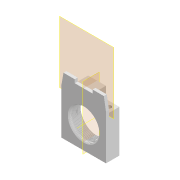
# Autodesk Inventor part: 30_Cube_Z_Focus_MGN_NEMA_adapter_RMS_bolted
Saved by Autodesk Inventor 2022 (Build 260153000, 153)
## iProperties
Created: 2021-04-25
Part Number: 30_Cube_Z_Focus_MGN_NEMA_adapter_RMS_bolted
Material: Generic
Document SubType Name: Modeling
Designer: diederichbenedict
Density: 1 g/cm^3
Appearance: Default
Author: diederichbenedict
Autodesk Inventor part; units mm, degrees
ref_plane "YZ Plane" through (0, 0, 0) normal (1, 0, 0) x (0, 1, 0)
ref_plane "XZ Plane" through (0, 0, 0) normal (0, 1, 0) x (-1, 0, 0)
ref_plane "XY Plane" through (0, 0, 0) normal (0, 0, 1) x (1, 0, 0)
ref_plane "Work Plane1" through (0, 0, 0) normal (0, 0, 1) x (1, 0, 0)
sketch "Sketch1" plane through (0, 0, 0) normal (0, 0, 1) x (1, 0, 0)
  circle A0 centre (6.843, -28.9967) radius 1.4 projected
  circle A1 centre (26.1569, -28.9967) radius 1.4 projected
  circle A2 centre (26.1569, -23.9967) radius 1.4 projected
  circle A3 centre (6.843, -23.9967) radius 1.4 projected
  line L0 (0.4643, -12) -> (0, -12) construction
  line L1 (3.1567, -14.6923) -> (0.4643, -12) construction
  line L2 (3.1567, -32.6831) -> (3.1567, -14.6923) construction
  line L3 (10.5294, -32.6831) -> (3.1567, -32.6831) projected
  line L4 (10.5294, -14.6923) -> (10.5294, -32.6831) construction
  line L5 (9, -11) -> (10.5294, -14.6923) construction
  line L6 (2.8, -11) -> (9, -11) construction
  line L7 (2.8, 0) -> (2.8, -11) construction
  line L8 (30.2, 0) -> (2.8, 0) construction
  line L9 (30.2, 0) -> (30.2, -11) construction
  line L10 (24, -11) -> (30.2, -11) construction
  line L11 (24, -11) -> (22.4706, -14.6923) construction
  line L12 (22.4706, -14.6923) -> (22.4706, -32.6831) construction
  line L13 (22.4706, -32.6831) -> (29.8433, -32.6831) projected
  line L14 (29.8433, -32.6831) -> (29.8433, -14.6923) construction
  line L15 (29.8433, -14.6923) -> (32.5357, -12) construction
  line L16 (33, -12) -> (32.5357, -12) construction
  line L17 (33, -12) -> (33, 5) construction
  line L18 (0, 5) -> (0, -12) construction
  circle A4 centre (16.4744, -46.03) radius 10 projected
  circle A5 centre (16.4744, -46.03) radius 12.5
  line L19 (31.4744, -31.03) -> (1.4744, -31.03) construction
  line L20 (1.4744, -31.03) -> (1.4744, -61.03) construction
  line L21 (1.4744, -61.03) -> (31.4744, -61.03) construction
  line L22 (31.4744, -61.03) -> (31.4744, -31.03) construction
  line L23 (31.4744, -31.03) -> (1.4744, -61.03) construction
  line L24 (1.4744, -31.03) -> (31.4744, -61.03) construction
  line L25 (31.4744, -61.03) -> (1.4744, -61.03)
  line L26 (1.4744, -61.03) -> (1.4744, -31.03)
  line L27 (1.4744, -31.03) -> (31.4744, -31.03)
  line L28 (31.4744, -31.03) -> (31.4744, -61.03)
  line L29 (31.4744, -61.03) -> (1.4744, -31.03) construction
  line L30 (1.4744, -61.03) -> (31.4744, -31.03) construction
  line L31 (1.4744, -31.03) -> (3.1567, -21.6555)
  line L32 (3.1567, -21.6555) -> (29.8433, -21.6555)
  line L33 (31.4744, -31.03) -> (29.8433, -21.6555)
  circle A6 centre (15.4444, 14.8) radius 2 projected
  line L34 (19.4444, 18.8) -> (33, 5) projected
  line L35 (11.4444, 18.8) -> (19.4444, 18.8) projected
  line L36 (0, 5) -> (11.4444, 18.8) projected
  circle A7 centre (3.9444, 3.3) radius 1.45 projected
  circle A8 centre (26.9444, 3.3) radius 1.45 projected
  point P0 (0, 0)
  dimension "d0" = 25
  dimension "d1" = 30
  dimension "d2" = 30
  constraints: 30 end point, 4 midpoint, 4 parallel, 3 perpendicular, 2 horizontal, 2 point on line, 1 centre point, 1 coincident
  measures "d0" diameter of A5
  measures "d1" distance of L21.end L20.end
  measures "d2" distance of L20.end L19.end
extrude "Extrusion1" add sketch "Sketch1" along normal blind 2 contours A0 | A1 | A2 | A3 | A5 | L25 L26 L27 L28 | L27 L31 L32 L33
sketch "Sketch2" plane through (0, 0, 0) normal (0, 0, -1) x (-1, 0, 0)
  circle A0 centre (-16.4744, -46.03) radius 12.5 projected
  circle A1 centre (-16.4744, -46.03) radius 10.5
  line L0 (0.4956, -63) -> (-33.4444, -63) projected
  circle A2 centre (-16.4744, -46.03) radius 12.5 projected
  arc A3 (-23.9744, -56.03) -> (-8.9744, -56.03) centre (-16.4744, -46.03) ccw
  arc A4 (-21.3847, -34.5348) -> (-28.8847, -47.5252) centre (-16.4744, -46.03) ccw
  arc A5 (-4.0642, -47.5252) -> (-11.5642, -34.5348) centre (-16.4744, -46.03) ccw
  point P0 (0, 0)
  dimension "d5" = 21
  constraints: 12 point on circle, 4 centre point, 2 coincident, 3 other
  measures "d5" diameter of A1
extrude "Extrusion2" add sketch "Sketch2" against normal up to surface (2 mm away)
sketch "Sketch3" plane through (0, 0, 0) normal (0, 0, -1) x (-1, 0, 0)
  line L0 (-30.5357, -14) -> (-24, -14) construction
  line L1 (-30.5357, -14) -> (-29.8433, -14.6923) construction
  line L2 (-29.8433, -14.6923) -> (-29.8433, -32.6831) construction
  line L3 (-29.8433, -32.6831) -> (-22.4706, -32.6831) projected
  line L4 (-22.4706, -32.6831) -> (-10.5294, -32.6831)
  line L5 (-10.5294, -32.6831) -> (-10.5294, -22.0651)
  line L6 (-10.5294, -22.0651) -> (-22.4706, -22.0651)
  line L7 (-22.4706, -22.0651) -> (-22.4706, -32.6831)
  line L8 (-1.4744, -31.03) -> (-3.1567, -21.6555) construction
  line L9 (-3.1567, -21.6555) -> (-29.8433, -21.6555) construction
  line L10 (-29.8433, -21.6555) -> (-31.4744, -31.03) construction
  line L11 (-31.4744, -31.03) -> (-31.4744, -61.03) construction
  line L12 (-31.4744, -61.03) -> (-1.4744, -61.03) projected
  line L13 (-1.4744, -61.03) -> (-1.4744, -31.03) construction
  line L14 (-31.4744, -32.6831) -> (-29.8433, -32.6831)
  line L15 (-3.1567, -32.6831) -> (-1.4744, -32.6831)
  line L16 (-31.4744, -61.03) -> (-1.4744, -61.03)
  line L17 (-1.4744, -61.03) -> (-1.4744, -32.6831)
  line L18 (-1.4744, -32.6831) -> (-31.4744, -32.6831)
  line L19 (-31.4744, -32.6831) -> (-31.4744, -61.03)
  circle A0 centre (-26.1569, -28.9967) radius 1.4 projected
  circle A1 centre (-26.1569, -23.9967) radius 1.4 projected
  line L20 (-24, -14) -> (-24, -11) projected
  line L21 (-22.4706, -32.6831) -> (-22.4706, -14.6923) projected
  line L22 (-22.4706, -14.6923) -> (-24, -11) projected
  circle A2 centre (-16.4256, -45.91) radius 10.6939 projected
  point P0 (0, 0)
  constraints: 20 end point, 4 parallel, 4 point on line, 2 horizontal, 2 perpendicular, 1 collinear
extrude "Extrusion4" add sketch "Sketch3" along normal blind 7 contours L3 L4 L18 L15 L17 L12 L19 L14 | L7 L6 L5 L4
sketch "Sketch4" plane through (3.1567, -21.6555, 0) normal (0, 1, 0) x (1, 0, 0)
  line L0 (-6.8596, 8.2929) -> (32.2101, 8.2929)
  line L1 (32.2101, 8.2929) -> (32.2101, -9.1799)
  line L2 (32.2101, -9.1799) -> (-6.8596, -9.1799)
  line L3 (-6.8596, -9.1799) -> (-6.8596, 8.2929)
  point P0 (-3.1567, 0)
  constraints: 8 end point, 2 parallel, 1 horizontal, 1 perpendicular
extrude "Extrusion5" cut sketch "Sketch4" against normal blind 1
sketch "Sketch5" plane through (0, 0, 2) normal (0, 0, 1) x (1, 0, 0)
  line L0 (30.0173, -22.6555) -> (2.9772, -22.6555) projected
  line L1 (2.9772, -22.6555) -> (1.4744, -31.03) projected
  line L2 (1.4744, -31.03) -> (1.4744, -61.03) projected
  line L3 (1.4744, -61.03) -> (31.4744, -61.03) projected
  line L4 (31.4744, -61.03) -> (31.4744, -31.03) projected
  line L5 (31.4744, -31.03) -> (30.0173, -22.6555) projected
  line L6 (10.5294, -20.3437) -> (22.4706, -20.3437)
  line L7 (22.4706, -20.3437) -> (22.4706, -24.9674)
  line L8 (22.4706, -24.9674) -> (10.5294, -24.9674)
  line L9 (10.5294, -24.9674) -> (10.5294, -20.3437)
  line L10 (10.5294, -22.6555) -> (22.4706, -22.6555) projected
  line L11 (10.5294, -20.3437) -> (22.4706, -24.9674) construction
  line L12 (22.4706, -20.3437) -> (10.5294, -24.9674) construction
  point P0 (0, 0)
  point P1 (16.5, -22.6555)
  constraints: 12 end point, 3 midpoint, 3 parallel, 1 perpendicular
extrude "Extrusion6" cut sketch "Sketch5" against normal through all contours L7 L8 L9 L0 | L0 L9 L6 L7
ref_plane "Work Plane2" through (16.4744, -61.03, 2) normal (1, 0, 0) x (0, 0, -1)
sketch "Sketch6" plane through (16.4744, -61.03, 2) normal (1, 0, 0) x (0, 0, -1)
  line L0 (0.0035, 5.17) -> (0.1535, 5.17)
  line L1 (0.0035, 5.17) -> (0.1535, 5.17) construction
  line L2 (0.1535, 5.17) -> (0.3562, 4.8189)
  line L3 (0.3562, 4.8189) -> (0.5062, 4.8189)
  line L4 (0.5062, 4.8189) -> (0.7089, 5.17)
  line L5 (0.7089, 5.17) -> (0.7089, 4.17)
  line L6 (0.7089, 4.17) -> (0.0035, 4.17)
  line L7 (0.0035, 4.17) -> (0.0035, 5.17)
  line L8 (-1.8, 15.12) -> (10.8, 15.12) projected
  point P0 (2, 61.03)
  point P1 (0, 0)
  dimension "d16" = 0.15
  dimension "d17" = 0
  dimension "d18" = 120
  dimension "d19" = 0.15
  dimension "d20" = 120
  dimension "d21" = 1
  dimension "d22" = 0.7054
  dimension "d33" = 9.95
  constraints: 16 end point, 3 perpendicular, 2 horizontal, 1 collinear, 1 parallel, 1 point on line
  measures "d16" distance of L0.start L0.end
  measures "d17" distance between parallel lines of L0 L1
  measures "d18" angle of L0 L2
  measures "d19" distance of L2.end L3.end
  measures "d20" angle of L4 L3
  measures "d21" distance of L4.end L5.end
  measures "d22" distance between parallel lines of L7 L5
  measures "d33" distance from line of L8 L4.end
coil "Coil1" sketch "Sketch6" operation add axis through (16.4744, -45.91, 0) along (0, 0, -1) pitch 0.7055 turns 12 hand right
sketch "Sketch11" plane through (16.4744, -61.03, 2) normal (1, 0, 0) x (0, 0, -1)
  line L0 (2.4721, 25.8139) -> (9, 25.8139) projected
  line L1 (-3.7827, 15.12) -> (16.1229, 15.12) projected
  line L2 (9.7248, 3.3163) -> (7.2115, 5.8296)
  line L3 (9.7248, 3.3163) -> (13.2792, 3.3163) construction
  line L4 (7.2115, 5.8296) -> (1.2979, 5.8296)
  line L5 (0, 30) -> (0, 0) projected
  line L6 (1.2979, 5.8296) -> (-0.9391, 3.5927)
  line L7 (-0.9391, 3.5927) -> (-0.9391, 12.5439)
  line L8 (-0.9391, 12.5439) -> (10.386, 12.5439)
  line L9 (10.386, 12.5439) -> (9.7248, 3.3163)
  point P0 (2, 61.03)
  point P1 (0, 12.5439)
  point P2 (0, 4.5318)
  dimension "d48" = 135
  dimension "d49" = 135
  constraints: 14 end point, 3 perpendicular, 1 equal length, 1 horizontal
  measures "d48" angle of L3 L2
  measures "d49" angle of L6 L4
revolve "Revolution1" cut sketch "Sketch11" angle 360 about axis through (16.4744, -45.91, 0) along (0, 0, -1) contours L2 L4 L6 L5 L8 L9
sketch "Sketch12" plane through (1.4744, -61.03, 2) normal (0, -1, 0) x (1, 0, 0)
  circle A0 centre (3.5, -5.5) radius 1.4 projected
  circle A1 centre (5, -17.7) radius 1.75 projected
  line L0 (9.9262, -23.9) -> (9.9262, 8.5) projected
  circle A2 centre (26.5, -5.5) radius 1.4 projected
hole "Hole1" at (4.9744, -61.03, -3.5) at (27.9744, -61.03, -3.5) direction (0, 1, 0) diameter 3 end through all counterbore diameter 6.5 counterbore depth 7
equation "\"d19\" = d16"
equation "\"d20\" = d18"
body "Solid1"
